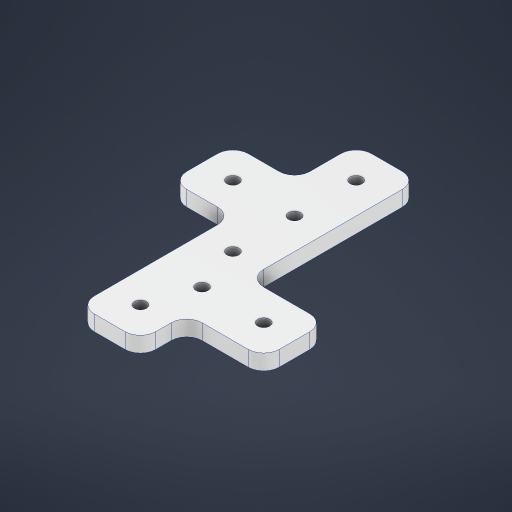
# Autodesk Inventor part: STRU_021_DVBSBracket2
Saved by Autodesk Inventor 2024.2 (Build 282272000, 272)
## iProperties
Created: 2024-07-28
Part Number: STRU_021_DVBSBracket2
Material: Aluminum 6061
Document SubType Name: Modeling
Designer: Bryan
Density: 2.7 g/cm^3
Appearance: Aluminum - Flat
Author: Bryan
Autodesk Inventor part; units mm, degrees
ref_plane "YZ Plane" through (0, 0, 0) normal (1, 0, 0) x (0, 1, 0)
ref_plane "XZ Plane" through (0, 0, 0) normal (0, 1, 0) x (-1, 0, 0)
ref_plane "XY Plane" through (0, 0, 0) normal (0, 0, 1) x (1, 0, 0)
sketch "Sketch1" plane through (0, 0, 0) normal (0, 1, 0) x (-1, 0, 0)
  line L0 (0, 6.35) -> (0, -6.35) construction
  line L1 (0, 0) -> (-6.35, 0) construction
  line L2 (0, -6.35) -> (0, -44.45) construction
  line L3 (0, -44.45) -> (12.7, -44.45) construction
  line L4 (0, -44.45) -> (0, -69.85) construction
  line L5 (-6.35, 0) -> (-31.75, 0) construction
  line L6 (0, 6.35) -> (0, 31.75) construction
  circle A0 centre (-6.35, 0) radius 2.4892
  circle A1 centre (-19.05, 0) radius 2.4892 construction
  circle A2 centre (-31.75, 0) radius 2.4892
  circle A3 centre (0, 31.75) radius 2.4892 construction
  circle A4 centre (0, 19.05) radius 2.4892
  circle A5 centre (0, 6.35) radius 2.4892 construction
  circle A6 centre (0, -6.35) radius 2.4892 construction
  circle A7 centre (0, -19.05) radius 2.4892
  circle A8 centre (0, -31.75) radius 2.4892 construction
  circle A9 centre (0, -44.45) radius 2.4892
  circle A10 centre (0, -57.15) radius 2.4892 construction
  circle A11 centre (0, -69.85) radius 2.4892
  circle A12 centre (12.7, -44.45) radius 2.4892 construction
  line L7 (12.7, -44.45) -> (38.1, -44.45) construction
  circle A13 centre (25.4, -44.45) radius 2.4892
  circle A14 centre (38.1, -44.45) radius 2.4892 construction
  line L8 (12.7, 31.75) -> (-12.7, 31.75)
  line L9 (12.7, 31.75) -> (12.7, -31.75)
  line L10 (12.7, -31.75) -> (38.1, -31.75)
  line L11 (38.1, -31.75) -> (38.1, -57.15)
  line L12 (38.1, -57.15) -> (12.7, -57.15)
  line L13 (12.7, -57.15) -> (12.7, -82.55)
  line L14 (12.7, -82.55) -> (-12.7, -82.55)
  line L15 (-12.7, -82.55) -> (-12.7, -12.7)
  line L16 (-12.7, -12.7) -> (-44.45, -12.7)
  line L17 (-44.45, -12.7) -> (-44.45, 12.7)
  line L18 (-44.45, 12.7) -> (-12.7, 12.7)
  line L19 (-12.7, 12.7) -> (-12.7, 31.75)
  point P0 (0, 31.75)
  point P1 (0, -82.55)
  point P2 (-44.45, 0)
  dimension "d0" = 12.7
  dimension "d1" = 6.35
  dimension "d2" = 38.1
  dimension "d3" = 12.7
  dimension "d4" = 25.4
  dimension "d5" = 25.4
  dimension "d6" = 25.4
  dimension "d7" = 4.9784
  dimension "d10" = 12.7
  dimension "d15" = 4.9784
  dimension "d18" = 12.7
  dimension "d23" = 4.9784
  dimension "d24" = 25.4
  dimension "d27" = 12.7
  dimension "d32" = 25.4
  dimension "d33" = 12.7
  dimension "d34" = 12.7
  dimension "d36" = 12.7
  constraints: 40 end point, 15 centre point, 12 horizontal, 11 vertical, 6 coincident, 6 midpoint, 3 perpendicular, 2 vertical alignment, 1 horizontal alignment, 24 other
  measures "d0" distance of L0.start L0.end
  measures "d1" distance of L1.start L1.end
  measures "d2" distance of L0.end L2.end
  measures "d3" distance of L2.end L3.end
  measures "d4" distance of L2.end L4.end
  measures "d5" distance of L1.end L5.end
  measures "d6" distance of L0.start L6.end
  measures "d7" diameter of A0
  measures "d10" distance of A0.centre A1.centre
  measures "d15" diameter of A3
  measures "d18" distance of A3.centre A4.centre
  measures "d23" diameter of A12
  measures "d24" distance of L7.start L7.end
  measures "d27" distance of L7.start A13.centre
  measures "d32" distance of L8.start L8.end
  measures "d33" distance from line of A4.centre L8
  measures "d34" distance from line of L17 L5.end
  measures "d36" distance from line of L14 L4.end
extrude "Extrusion1" add sketch "Sketch1" along normal blind 6.35
fillet "Fillet1" radius 6.35 12 edges at (-12.7, 3.175, 31.75) (12.7, 3.175, 31.75) (12.7, 3.175, 12.7) (-12.7, 3.175, -31.75) (-38.1, 3.175, -31.75) (-38.1, 3.175, -57.15) (-12.7, 3.175, -57.15) (-12.7, 3.175, -82.55) (12.7, 3.175, -82.55) (44.45, 3.175, -12.7) (12.7, 3.175, -12.7) (44.45, 3.175, 12.7)
body "Solid1"
